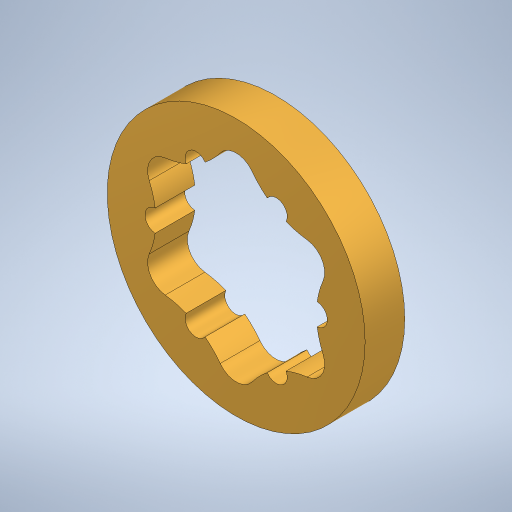
# Autodesk Inventor part: Brass Gryo
Saved by Autodesk Inventor 2023.2 (Build 272271000, 271)
## iProperties
Created: 2023-06-11
Part Number: Brass Gryo
Material: Brass, Soft Yellow
Document SubType Name: Modeling
Designer: Nathan Cai
Density: 8.47 g/cm^3
Appearance: Brass - Satin
Mass: 36.4777 g
Surface Area: 28.7122 cm^2
Volume: 4.30669 cm^3
Brass_ID: 1.250 in
Author: Nathan Cai
Autodesk Inventor part; units mm, degrees
ref_plane "YZ Plane" through (0, 0, 0) normal (1, 0, 0) x (0, 1, 0)
ref_plane "XZ Plane" through (0, 0, 0) normal (0, 1, 0) x (-1, 0, 0)
ref_plane "XY Plane" through (0, 0, 0) normal (0, 0, 1) x (1, 0, 0)
sketch "Sketch1" plane through (0, 0, 0) normal (0, 0, 1) x (1, 0, 0)
  circle A0 centre (0, 0) radius 20.6375
  circle A1 centre (0, 0) radius 7.9375 construction
  circle A2 centre (0, 0) radius 15.875
  line L0 (0, 0) -> (0, 20.6375) construction
  circle A3 centre (0, 0) radius 3.175 construction
  circle A4 centre (0, 12.7) radius 3.175
  line L1 (0, 12.7) -> (10.9985, 6.35) construction
  line L2 (10.9985, 6.35) -> (10.9985, -6.35) construction
  line L3 (10.9985, -6.35) -> (0, -12.7) construction
  line L4 (0, -12.7) -> (-10.9985, -6.35) construction
  line L5 (-10.9985, -6.35) -> (-10.9985, 6.35) construction
  line L6 (-10.9985, 6.35) -> (0, 12.7) construction
  circle A5 centre (10.9985, 6.35) radius 3.175
  arc A6 (2.5548, 14.5851) -> (11.3536, 9.5051) centre (12.7741, 22.1254) ccw
  arc A7 (-11.3536, 9.5051) -> (-2.5548, 14.5851) centre (-12.7741, 22.1254) ccw
  circle A8 centre (0, 12.7) radius 3.175
  arc A9 (-13.9085, -5.08) -> (-13.9085, 5.08) centre (-25.5482, 0) ccw
  circle A10 centre (-10.9985, 6.35) radius 3.175
  arc A11 (-2.5548, -14.5851) -> (-11.3536, -9.5051) centre (-12.7741, -22.1254) ccw
  circle A12 centre (-10.9985, -6.35) radius 3.175
  arc A13 (11.3536, -9.5051) -> (2.5548, -14.5851) centre (12.7741, -22.1254) ccw
  circle A14 centre (0, -12.7) radius 3.175
  arc A15 (13.9085, 5.08) -> (13.9085, -5.08) centre (25.5482, 0) ccw
  circle A16 centre (10.9985, -6.35) radius 3.175
  circle A17 centre (6.4241, -11.1269) radius 1.7526
  circle A18 centre (12.8482, 0) radius 1.7526
  circle A19 centre (6.4241, 11.1269) radius 1.7526
  circle A20 centre (-6.4241, 11.1269) radius 1.7526
  circle A21 centre (-12.8482, 0) radius 1.7526
  circle A22 centre (-6.4241, -11.1269) radius 1.7526
  point P0 (13.9085, 5.08)
  point P1 (11.3536, -9.5051)
  point P2 (-2.5548, -14.5851)
  point P3 (-13.9085, -5.08)
  point P4 (-11.3536, 9.5051)
  point P5 (-2.5548, 14.5851)
  point P6 (12.9691, 1.7484)
  point P7 (12.9691, -1.7484)
  point P8 (7.9987, -10.3574)
  point P9 (4.9704, -12.1058)
  point P10 (-4.9704, -12.1058)
  point P11 (-7.9987, -10.3574)
  point P12 (-12.9691, -1.7484)
  point P13 (-12.9691, 1.7484)
  point P14 (-7.9987, 10.3574)
  point P15 (-4.9704, 12.1058)
  point P16 (4.9704, 12.1058)
  point P17 (7.9987, 10.3574)
  dimension "d0" = 41.275
  dimension "d13" = 6.35
  dimension "d14" = 6.35
  dimension "d1" = 15.875
  dimension "d4" = 6.35
  dimension "d15" = 12.7
  dimension "d18" = 360
  dimension "d20" = 3.5052
  dimension "d23" = 360
  dimension "Brass_ID" = 31.75
  constraints: 15 centre point, 14 end point, 13 point on circle, 6 coincident, 1 point on line, 1 vertical, 1 vertical alignment, 89 other
  measures "d1" diameter of A1
  measures "d4" diameter of A3
  measures "d15" radius of A6
  measures "d20" diameter of A17
  measures "Brass_ID" diameter of A2
extrude "Extrusion1" add sketch "Sketch1" along normal blind 6.35 contours A0 | A2 A16 A15 A18 A5 | A5 A6 A19 A4 A2 | A2 A14 A13 A17 A16 | A4 A7 A20 A10 A2 | A2 A12 A11 A22 A14 | A10 A9 A21 A12 A2
equation "\"d0\" = Brass_OD"
equation "\"Brass_OD\" = 41.275"
body "Solid1"
